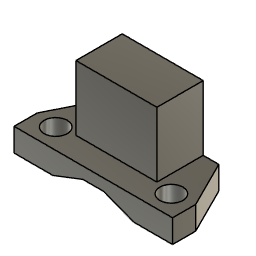
hallEffectHolder (Autodesk Fusion 360 design; units mm, degrees)
Autodesk Fusion 360 part; units mm, degrees
sketch "mainBase" plane through (0, 0, 0) normal (0, 0, 1) x (1, 0, 0)
  line L0 (0, 0) -> (13.7, 0)
  line L1 (13.7, 0) -> (13.7, 6)
  line L2 (13.7, 6) -> (0, 6)
  line L3 (0, 6) -> (0, 0)
  line L4 (0, 0) -> (6.85, 0)
  line L5 (6.85, 0) -> (6.85, 1.75)
  line L6 (6.85, 1.75) -> (1.85, 1.75)
  line L7 (6.85, 1.75) -> (11.85, 1.75)
  line L8 (0, 6) -> (6.85, 6)
  circle A0 centre (1.85, 1.75) radius 1
  circle A1 centre (11.85, 1.75) radius 1
  line L9 (6.85, 6) -> (3.35, 6)
  line L10 (3.35, 6) -> (3.35, 2)
  line L11 (3.35, 2) -> (6.85, 2)
  line L12 (6.85, 2) -> (6.85, 6)
  line L13 (6.85, 6) -> (10.35, 6)
  line L14 (10.35, 6) -> (10.35, 2)
  line L15 (10.35, 2) -> (6.85, 2)
  line L16 (6.85, 2) -> (6.85, 6)
  dimension "d9" = 6
  dimension "d10" = 13.7
  dimension "d11" = 6.85
  dimension "d12" = 1.75
  dimension "d13" = 5
  dimension "d14" = 5
  dimension "d15" = 6.85
  dimension "d17" = 2
  dimension "d18" = 2
  dimension "d19" = 4
  dimension "d20" = 3.5
  dimension "d21" = 4
  dimension "d22" = 3.5
  constraint horizontal L0
  constraint vertical L1
  constraint horizontal L2
  constraint vertical L3
  constraint coincident L0.start L3.end
  constraint perpendicular L3 L4
  constraint perpendicular L0 L5
  constraint perpendicular L5 L6
  constraint perpendicular L5 L7
  constraint perpendicular L3 L8
  constraint coincident L6.end A0.centre
  constraint coincident L7.end A1.centre
  constraint horizontal L9
  constraint vertical L10
  constraint horizontal L11
  constraint vertical L12
  constraint horizontal L13
  constraint vertical L14
  constraint horizontal L15
  constraint vertical L16
  measures "d9" distance of L0.start L2.end
  measures "d10" distance of L0.start L0.end
  measures "d11" distance of L0.start L4.end
  measures "d12" distance of L4.end L5.end
  measures "d13" distance of L5.end L6.end
  measures "d14" distance of L5.end L7.end
  measures "d15" distance of L2.end L8.end
  measures "d17" diameter of A0
  measures "d18" diameter of A1
  measures "d19" distance of L8.end L11.end
  measures "d20" distance of L10.end L11.end
  measures "d21" distance of L8.end L11.end
  measures "d22" distance of L14.end L11.end
extrude "Extrude1" add sketch "mainBase" along normal blind 7.6 contours L2 L8 L9 L10 L11 L12 L16 | L2 L12 L13 L14 L15 L16
shell "Shell1" thickness 1 removed faces 1 at (8.0167, 4.6667, 0)
extrude "Extrude2" add sketch "mainBase" along normal blind 2 contours L0 L1 L2 L3 L4 L8 L10 L11 L14 L15
sketch "hallCutOut" plane through (0, 0, 0) normal (0, 0, 1) x (1, 0, 0)
  line L0 (0, 6) -> (6.85, 6)
  line L1 (6.85, 6) -> (6.85, 2)
  line L2 (6.85, 2) -> (3.35, 2)
  line L3 (3.35, 2) -> (3.35, 4)
  line L4 (6.85, 2) -> (6.85, 3)
  line L5 (6.85, 3) -> (5.95, 3)
  line L6 (5.95, 3) -> (3.35, 4)
  line L7 (6.85, 3) -> (7.75, 3)
  line L8 (6.85, 2) -> (10.35, 2)
  line L9 (10.35, 2) -> (10.35, 4)
  line L10 (10.35, 4) -> (7.75, 3)
  line L11 (7.75, 3) -> (9.35, 3)
  line L12 (9.35, 3) -> (9.35, 3.6154)
  line L13 (5.95, 3) -> (4.35, 3)
  line L14 (4.35, 3) -> (4.35, 3.6154)
  line L15 (6.85, 5) -> (8.95, 5)
  line L16 (8.95, 5) -> (8.95, 3)
  line L17 (8.95, 3) -> (6.85, 3)
  line L18 (6.85, 3) -> (6.85, 5)
  line L19 (6.85, 5) -> (4.75, 5)
  line L20 (4.75, 5) -> (4.75, 3)
  line L21 (4.75, 3) -> (6.85, 3)
  line L22 (6.85, 3) -> (6.85, 5)
  line L23 (9.35, 3) -> (4.35, 3)
  line L24 (4.35, 3) -> (4.35, 5)
  line L25 (4.35, 5) -> (9.35, 5)
  line L26 (9.35, 5) -> (9.35, 3)
  dimension "d31" = 6.85
  dimension "d32" = 4
  dimension "d33" = 3.5
  dimension "d34" = 2
  dimension "d35" = 1
  dimension "d36" = 0.9
  dimension "d37" = 0.9
  dimension "d38" = 3.5
  dimension "d39" = 2
  dimension "d59" = 2.1
  constraint horizontal L0
  constraint perpendicular L0 L1
  constraint perpendicular L1 L2
  constraint perpendicular L2 L3
  constraint perpendicular L2 L4
  constraint perpendicular L1 L5
  constraint perpendicular L1 L7
  constraint perpendicular L4 L8
  constraint perpendicular L8 L9
  constraint parallel L7 L11
  constraint coincident L10 L12.end
  constraint perpendicular L11 L12
  constraint perpendicular L1 L13
  constraint coincident L6 L14.end
  constraint perpendicular L13 L14
  constraint horizontal L15
  constraint vertical L16
  constraint horizontal L17
  constraint vertical L18
  constraint coincident L1 L15.start
  constraint horizontal L19
  constraint vertical L20
  constraint horizontal L21
  constraint vertical L22
  constraint coincident L13 L20.end
  constraint horizontal L23
  constraint vertical L24
  constraint horizontal L25
  constraint vertical L26
  measures "d31" distance of L0.start L0.end
  measures "d32" distance of L0.end L1.end
  measures "d33" distance of L1.end L2.end
  measures "d34" distance of L2.end L3.end
  measures "d35" distance of L1.end L4.end
  measures "d36" distance of L4.end L5.end
  measures "d37" distance of L4.end L7.end
  measures "d38" distance of L1.end L8.end
  measures "d39" distance of L8.end L9.end
  measures "d59" distance of L15.start L15.end
extrude "Extrude3" add sketch "hallCutOut" along normal blind 6.6 contours L6 L13 L20 L21 L23 | L10 L11 L16 L17 L23 | L10 L11 L12 L16 L23 L26 | L6 L13 L14 L20 L23 L24
sketch "wireCutOut" plane through (0, 0, 0) normal (0, -1, 0) x (1, 0, 0)
  line L0 (0, 0) -> (13.7, 0)
  line L1 (13.7, 0) -> (13.7, 2)
  line L2 (13.7, 2) -> (0, 2)
  line L3 (0, 2) -> (0, 0)
  line L4 (0, 0) -> (6.85, 0)
  line L5 (6.85, 0) -> (6.85, 1)
  line L6 (6.85, 1) -> (5.95, 1)
  line L7 (6.85, 1) -> (7.75, 1)
  line L8 (6.85, 0) -> (13.7, 0)
  line L9 (6.85, 0) -> (10.35, 0)
  line L10 (6.85, 0) -> (3.35, 0)
  line L11 (7.75, 1) -> (10.35, 0)
  line L12 (5.95, 1) -> (3.35, 0)
  dimension "d42" = 6.85
  dimension "d43" = 1
  dimension "d44" = 0.9
  dimension "d45" = 0.9
  dimension "d46" = 6.85
  dimension "d47" = 3.5
  dimension "d48" = 3.5
  constraint coincident L0.start L3.end
  constraint perpendicular L3 L4
  constraint perpendicular L4 L5
  constraint perpendicular L5 L6
  constraint perpendicular L5 L7
  constraint perpendicular L5 L8
  constraint perpendicular L5 L9
  constraint perpendicular L5 L10
  measures "d42" distance of L0.start L4.end
  measures "d43" distance of L4.end L5.end
  measures "d44" distance of L5.end L6.end
  measures "d45" distance of L5.end L7.end
  measures "d46" distance of L4.end L0.end
  measures "d47" distance of L4.end L9.end
  measures "d48" distance of L4.end L10.end
extrude "Extrude4" cut sketch "wireCutOut" against normal blind 5 contours L0 L4 L5 L6 L10 L12 | L0 L5 L7 L8 L9 L11
sketch "cutOut" plane through (0, 0, 0) normal (0, 0, 1) x (1, 0, 0)
  line L0 (0, 0) -> (13.7, 0)
  line L1 (13.7, 0) -> (13.7, 6)
  line L2 (13.7, 6) -> (0, 6)
  line L3 (0, 6) -> (0, 0)
  line L4 (13.7, 0) -> (13.7, 2)
  line L5 (0, 0) -> (0, 2)
  line L6 (0, 6) -> (2, 6)
  line L7 (13.7, 6) -> (11.7, 6)
  line L8 (0, 2) -> (2, 6)
  line L9 (13.7, 2) -> (11.7, 6)
  dimension "d51" = 6
  dimension "d52" = 13.7
  dimension "d53" = 2
  dimension "d54" = 2
  dimension "d55" = 2
  dimension "d56" = 2
  constraint horizontal L0
  constraint vertical L1
  constraint horizontal L2
  constraint vertical L3
  constraint coincident L0.start L3.end
  constraint perpendicular L0 L4
  constraint perpendicular L0 L5
  constraint coincident L2 L6.end
  constraint perpendicular L1 L7
  measures "d51" distance of L0.start L2.end
  measures "d52" distance of L0.start L0.end
  measures "d53" distance of L0.end L4.end
  measures "d54" distance of L0.start L5.end
  measures "d55" distance of L1.end L7.end
  measures "d56" distance of L2.end L6.end
extrude "Extrude5" cut sketch "cutOut" along normal blind 2 contours L2 L3 L6 L8 | L1 L2 L7 L9
extrude "Extrude6" add sketch "hallCutOut" along normal blind 7.6 contours L10 L16 L25 L26 | L6 L20 L24 L25
extrude "Extrude7" cut sketch "wireCutOut" against normal blind 5 contours L0 L4 L5 L6 L10 L12 | L0 L5 L7 L8 L9 L11
equation "baseLength = 6 mm"
equation "baseWidth = 13.7 mm"
equation "mountingCircleToMountingCircle = 10 mm"
equation "mountingHoleFromEdge = 1.75 mm"
equation "hallEffectWidth = 7 mm"
equation "hallEffectLength = 4 mm"
equation "hallEffectHeight = 7.6 mm"
equation "baseHeight = 2 mm"
equation "d9 = baseLength"
equation "d10 = baseWidth"
equation "d11 = baseWidth / 2"
equation "d12 = mountingHoleFromEdge"
equation "d13 = mountingCircleToMountingCircle / 2"
equation "d14 = mountingCircleToMountingCircle / 2"
equation "d15 = baseWidth / 2"
equation "screwHole = 2 mm"
equation "d17 = screwHole"
equation "d18 = screwHole"
equation "d19 = hallEffectLength"
equation "d20 = hallEffectWidth / 2"
equation "d21 = hallEffectLength"
equation "d22 = hallEffectWidth / 2"
equation "d23 = hallEffectHeight"
equation "hallEffectThickness = 1 mm"
equation "d26 = hallEffectThickness"
equation "d27 = baseHeight"
equation "traingleHeight = 2 mm"
equation "hallEffectMiddleDist = 1.8 mm"
equation "d31 = baseWidth / 2"
equation "d32 = hallEffectLength"
equation "d33 = hallEffectWidth / 2"
equation "d34 = traingleHeight"
equation "d35 = hallEffectThickness"
equation "d36 = hallEffectMiddleDist / 2"
equation "d37 = hallEffectMiddleDist / 2"
equation "d38 = hallEffectWidth / 2"
equation "d39 = traingleHeight"
equation "d40 = hallEffectHeight - hallEffectThickness"
equation "d42 = baseWidth / 2"
equation "d43 = hallEffectThickness"
equation "d44 = hallEffectMiddleDist / 2"
equation "d45 = hallEffectMiddleDist / 2"
equation "d46 = baseWidth / 2"
equation "d47 = hallEffectWidth / 2"
equation "d48 = hallEffectWidth / 2"
equation "d49 = -( baseLength - hallEffectThickness )"
equation "d51 = baseLength"
equation "d52 = baseWidth"
equation "d53 = baseLength / 3"
equation "d54 = baseLength / 3"
equation "d57 = baseHeight"
equation "d60 = hallEffectHeight"
equation "d62 = -hallEffectLength - hallEffectThickness"
